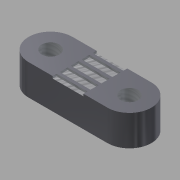
# Autodesk Inventor part: belt-clamp
Saved by Autodesk Inventor 2011 SP2 (Build 150309200, 309)
## iProperties
Created: 2012-10-08
Part Number: belt-clamp
Document SubType Name: Modeling
Designer: Greg Pavlik
Density: 1 g/cm^3
Author: Greg Pavlik
Autodesk Inventor part; units mm, degrees
ref_plane "YZ Plane" through (0, 0, 0) normal (1, 0, 0) x (0, 1, 0)
ref_plane "XZ Plane" through (0, 0, 0) normal (0, 1, 0) x (-1, 0, 0)
ref_plane "XY Plane" through (0, 0, 0) normal (0, 0, 1) x (1, 0, 0)
sketch "Sketch1" plane through (0, 0, 0) normal (0, 0, 1) x (1, 0, 0)
  arc A0 (0, 5) -> (0, -5) centre (0, 0) ccw
  line L0 (0, 0) -> (18, 0) construction
  line L1 (18, 5) -> (0, 5)
  line L2 (0, -5) -> (18, -5)
  arc A1 (18, -5) -> (18, 5) centre (18, 0) ccw
  dimension "d0" = 5
  dimension "d1" = 18
  constraints: 6 end point, 4 point on circle, 4 tangent, 2 centre point, 2 coincident, 1 horizontal, 1 parallel
  measures "d0" radius of A0
  measures "d1" distance of L0.end point (0, 0)
extrude "Extrusion1" add sketch "Sketch1" along normal blind 7
sketch "Sketch2" plane through (0, 0, 7) normal (0, 0, 1) x (1, 0, 0)
  arc A0 (18, -5) -> (18, 5) centre (18, 0) ccw projected
  arc A1 (0, 5) -> (0, -5) centre (0, 0) ccw projected
  constraints: 2 coincident
hole "Hole1" at (0, 0, 7) at (18, 0, 7) direction (0, 0, -1) diameter 4 end through all
sketch "Sketch3" plane through (0, 0, 7) normal (0, 0, 1) x (1, 0, 0)
  line L0 (0, 5) -> (18, 5) projected
  line L1 (18, -5) -> (0, -5) projected
  line L2 (12.5, 0.9) -> (5.5, 0.9)
  line L3 (5.5, 0.9) -> (5.5, -0.9)
  line L4 (5.5, -0.9) -> (12.5, -0.9)
  line L5 (12.5, -0.9) -> (12.5, 0.9)
  line L6 (12.5, -1.6) -> (5.5, -1.6)
  line L7 (5.5, -1.6) -> (5.5, -3.4)
  line L8 (5.5, -3.4) -> (12.5, -3.4)
  line L9 (12.5, -3.4) -> (12.5, -1.6)
  line L10 (12.5, 1.6) -> (5.5, 1.6)
  line L11 (5.5, 1.6) -> (5.5, 3.4)
  line L12 (5.5, 3.4) -> (12.5, 3.4)
  line L13 (12.5, 3.4) -> (12.5, 1.6)
  line L14 (5.5, 4.1) -> (12.5, 4.1)
  line L15 (12.5, 4.1) -> (12.5, 5)
  line L16 (12.5, 5) -> (5.5, 5)
  line L17 (5.5, 5) -> (5.5, 4.1)
  line L18 (12.5, -4.1) -> (5.5, -4.1)
  line L19 (5.5, -4.1) -> (5.5, -5)
  line L20 (5.5, -5) -> (12.5, -5)
  line L21 (12.5, -5) -> (12.5, -4.1)
  line L22 (9, 5) -> (9, -5) construction
  line L23 (9, 5) -> (9, 7.1624) construction
  line L24 (12.5, 3.4) -> (12.5, 4.1) construction
  line L25 (12.5, 1.6) -> (12.5, 0.9) construction
  line L26 (12.5, -0.9) -> (12.5, -1.6) construction
  line L27 (12.5, -3.4) -> (12.5, -4.1) construction
  point P0 (9, 4.1)
  dimension "d11" = 7
  dimension "d12" = 0.7
  dimension "d13" = 1.8
  constraints: 52 end point, 21 collinear, 12 parallel, 5 horizontal, 5 perpendicular, 4 midpoint, 1 point on line
  measures "d11" distance between parallel lines of L15 L17
  measures "d12" distance of L4.end L6.start
  measures "d13" distance of L4.end L2.start
extrude "Extrusion2" cut sketch "Sketch3" against normal blind 0.5
body "Solid1"
